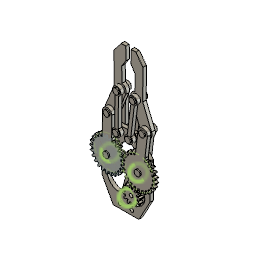
Robotic+Gripper (Autodesk Fusion 360 design; units mm, degrees)
description: Spur Gear; Module: 1.125000; Num Teeth: 24; Pressure Angle: 20.000000; Backlash: 0.00 mm
description: Spur Gear; Module: 1.100000; Num Teeth: 12; Pressure Angle: 20.000000; Backlash: 0.00 mm
Autodesk Fusion 360 part; units mm, degrees
note: some values were not read from the file. Chosen so that the rebuilt part matches the saved one: a direction. Set by a fixed rule: which sketch regions a step uses.
(part 1 of 5)
sketch "Sketch1" plane through (0, 0, 0) normal (0, 0, 1) x (1, 0, 0)
  line L0 (0, -5) -> (22, -5)
  arc A0 (22, -5) -> (22, 5) centre (22, 0) ccw
  line L1 (22, 5) -> (0, 5)
  arc A1 (0, 5) -> (0, -5) centre (0, 0) ccw
  line L2 (0, 0) -> (22, 0) construction
  circle A2 centre (0, 0) radius 1.5
  circle A3 centre (22, 0) radius 1.5
  line L3 (51.4959, 17.929) -> (55.4376, 8.3418)
  line L4 (55.4376, 8.3418) -> (23.9013, -4.6244)
  line L5 (51.4959, 17.929) -> (20.05, 5)
  line L6 (44.0768, 14.8786) -> (53.863, 12.1717)
  line L7 (39.0014, 5.4117) -> (26.978, 0.4683)
  line L8 (39.0014, 5.4117) -> (45.3296, 4.1859)
  dimension "d1" = 22
  dimension "d2" = 10
  dimension "d3" = 3
  dimension "d4" = 3
  dimension "d7" = 1.95
  dimension "d8" = 157.65
  dimension "d9" = 34
  dimension "d10" = 13
  constraint tangent L0 A0
  constraint tangent A0 L1
  constraint parallel L0 L1
  constraint tangent L1 A1
  constraint tangent L0 A1
  constraint horizontal L2
  constraint coincident A1.centre L2.start
  constraint concentric A1 A2
  constraint concentric A0 A3
  constraint coincident A0 L4.end
  constraint tangent A0 L4
  constraint perpendicular L3 L4
  constraint coincident L1 L5.end
  constraint perpendicular L3 L5
  constraint coincident L5 L6.start
  constraint coincident L3 L6.end
  constraint coincident A0 L7.end
  constraint perpendicular L3 L7
  constraint coincident L4 L8.end
  measures "d1" distance of A1.centre A0.centre
  measures "d2" diameter of A0
  measures "d3" diameter of A2
  measures "d4" diameter of A3
  measures "d7" horizontal distance of A0.centre L5.end
  measures "d8" angle of L1 L5
  measures "d9" distance of L3.start L5.end
  measures "d10" distance of L7.start L7.end
extrude "Extrude1" add sketch "Sketch1" along normal blind 3 contours L0 A0 L1 A1 | A0 L1 L3 L4 L5 L6 L7 L8 makes body 1 in component "Gripper (1)"
sketch "Sketch2" plane through (0, 0, 0) normal (0, 0, 1) x (1, 0, 0)
  circle A0 centre (5, 10) radius 1.5
  circle A1 centre (5, 10) radius 3.5
  line L0 (5, 10) -> (36, 10)
  circle A2 centre (36, 10) radius 1.5
  circle A3 centre (36, 10) radius 3.5
  line L1 (8.1623, 11.5) -> (32.8377, 11.5)
  line L2 (8.1623, 8.5) -> (32.8377, 8.5)
  dimension "d13" = 3
  dimension "d14" = 7
  dimension "d15" = 3
  dimension "d16" = 7
  dimension "d17" = 31
  dimension "d18" = 1.5
  constraint concentric A0 A1
  constraint coincident A0.centre A1.centre
  constraint horizontal L0
  constraint coincident L0.end A2.centre
  constraint concentric A2 A3
  constraint coincident A1 L1.start
  constraint coincident A3 L1.end
  constraint horizontal L1
  constraint symmetric L0 L1.start L2.start
  constraint symmetric L0 L1.end L2.end
  measures "d13" diameter of A0
  measures "d14" diameter of A1
  measures "d15" diameter of A2
  measures "d16" diameter of A3
  measures "d17" distance of A0.centre L0.end
  measures "d18" distance of L0 L1
extrude "Extrude1'" add sketch "Sketch2" along normal blind 3 separate body makes body 2 in component "Connecting rod"
sketch "Sketch3" plane through (0, 0, 0) normal (0, 0, 1) x (1, 0, 0)
  line L0 (0, 0) -> (0, 62) construction
  line L1 (0, 62) -> (-7.9898, 62)
  line L2 (-7.9898, 62) -> (-20.5, 47.8997)
  line L3 (-20.5, 47.8997) -> (-20.5, 17.5997)
  line L4 (-11, 0) -> (0, 0)
  line L5 (-20.5, 17.5997) -> (-11, 0)
  circle A0 centre (-5.2398, 58) radius 1.5
  circle A1 centre (-13.5, 37.5997) radius 1.5
  circle A2 centre (-5, 4) radius 1.5
  circle A3 centre (13.5, 37.5997) radius 1.5
  line L6 (20.5, 17.5997) -> (11, 0)
  circle A4 centre (5.2398, 58) radius 1.5
  line L7 (7.9898, 62) -> (20.5, 47.8997)
  line L8 (20.5, 47.8997) -> (20.5, 17.5997)
  line L9 (11, 0) -> (0, 0)
  line L10 (0, 62) -> (7.9898, 62)
  circle A5 centre (5, 4) radius 1.5
  circle A6 centre (7.5, 17.5997) radius 8.5
  line L11 (20.5, 17.5997) -> (0, 17.5997) construction
  dimension "d21" = 62
  dimension "d22" = 11
  dimension "d23" = 20
  dimension "d24" = 20.5
  dimension "d25" = 30.3
  dimension "d26" = 18.85
  dimension "d27" = 3
  dimension "d28" = 4
  dimension "d29" = 2.75
  dimension "d30" = 3
  dimension "d31" = 3
  dimension "d32" = 7
  dimension "d33" = 10.3
  dimension "d34" = 4
  dimension "d35" = 6
  dimension "d36" = 17
  dimension "d37" = 13
  constraint coincident L0.start L4.end
  constraint vertical L0
  constraint perpendicular L0 L1
  constraint perpendicular L1 L3
  constraint perpendicular L0 L4
  constraint symmetric L4.end L0 L9.end
  constraint symmetric L1.start L0 L10.start
  constraint symmetric L0 L1.end L7.start
  constraint symmetric L0 L2.end L7.end
  constraint symmetric L0 L3.end L6.start
  constraint symmetric L0 L4.start L6.end
  constraint symmetric L0 L4.end L9.end
  constraint symmetric L0 A0 A4
  constraint symmetric L0 A1 A3
  constraint symmetric L0 A2 A5
  constraint coincident L0 L11.end
  constraint perpendicular L0 L11
  measures "d21" distance of L0.start L0.end
  measures "d22" distance of L4.start L0.start
  measures "d23" distance of L3.end L4.start
  measures "d24" distance of L0 L3
  measures "d25" distance of L2.end L3.end
  measures "d26" distance of L1.end L2.end
  measures "d27" diameter of A0
  measures "d28" distance of L1 A0.centre
  measures "d29" horizontal distance of L1.end A0.centre
  measures "d30" diameter of A1
  measures "d31" diameter of A2
  measures "d32" distance of L3 A1.centre
  measures "d33" vertical distance of L2.end A1.centre
  measures "d34" distance of L4 A2.centre
  measures "d35" horizontal distance of L4.start A2.centre
  measures "d36" diameter of A6
  measures "d37" distance of L6.start A6.centre
extrude "Extrude1''" add sketch "Sketch3" along normal blind 3 separate body makes body 3 in component "Component"
sketch "Sketch4" plane through (0, 0, 3) normal (0, 0, 1) x (1, 0, 0)
  circle A0 centre (5, 4) radius 1.5
  circle A1 centre (7.5, 17.5997) radius 8.5
  circle A2 centre (-13.5, 37.5997) radius 1.5
  circle A3 centre (-5, 4) radius 1.5
  circle A4 centre (13.5, 37.5997) radius 1.5
  circle A5 centre (5.2398, 58) radius 1.5
  circle A6 centre (-5.2398, 58) radius 1.5
  line L0 (-7.9898, 62) -> (-20.5, 47.8997)
  line L1 (-20.5, 47.8997) -> (-20.5, 17.5997)
  line L2 (-20.5, 17.5997) -> (-11, 0)
  line L3 (-11, 0) -> (11, 0)
  line L4 (11, 0) -> (20.5, 17.5997)
  line L5 (20.5, 17.5997) -> (20.5, 47.8997)
  line L6 (20.5, 47.8997) -> (7.9898, 62)
  line L7 (7.9898, 62) -> (-7.9898, 62)
  spline S0 degree 5 poles (-12.9887, 25.9698) (-12.8812, 26.0083) (-12.6712, 26.1424) (-12.369, 26.5664) (-11.9726, 27.7138) (-11.4084, 30.1864) (-10.6796, 33.5496) (-9.6904, 37.5033) (-8.3597, 41.6551) (-6.6383, 45.5821) (-4.523, 48.8897) (-2.0756, 51.2778) (0.5698, 52.5846) (3.2369, 52.7612) (5.73, 51.8583) (7.8603, 50.0084) (9.4696, 47.4098) (10.4581, 44.3118) (10.8014, 40.9955) (10.5337, 37.7435) (9.7361, 34.8098) (8.5231, 32.3916) (7.0294, 30.5968) (5.398, 29.4192) (3.7666, 28.6961) (2.255, 28.1207) (0.9516, 27.3511) (-0.1001, 26.0957) (-0.9153, 24.2102) (-1.5814, 21.787) (-2.2274, 19.0805) (-2.9952, 16.4345) (-4.0102, 14.2098) (-5.352, 12.7108) (-7.0248, 12.1143) (-8.9268, 12.3927) (-10.8888, 13.3779) (-12.7158, 14.8289) (-14.2263, 16.4978) (-15.2944, 18.1976) (-15.8878, 19.8639) (-16.0433, 21.491) (-15.8437, 23.0636) (-15.3956, 24.5094) (-14.8046, 25.5948) (-14.1624, 26.0841) (-13.6639, 26.001) (-13.3163, 25.9113) (-13.0962, 25.9312) (-12.9887, 25.9698) knots 0 0 0 0 0 0 0.022222 0.044444 0.066667 0.088889 0.111111 0.133333 0.155556 0.177778 0.2 0.222222 0.244444 0.266667 0.288889 0.311111 0.333333 0.355556 0.377778 0.4 0.422222 0.444444 0.466667 0.488889 0.511111 0.533333 0.555556 0.577778 0.6 0.622222 0.644444 0.666667 0.688889 0.711111 0.733333 0.755556 0.777778 0.8 0.822222 0.844444 0.866667 0.888889 0.911111 0.933333 0.955556 0.977778 1 1 1 1 1 1
  point P0 (-5, 47.9245)
  point P1 (9, 47.9245)
  point P2 (6, 29.9245)
  point P3 (-0.0238, 25.9698)
  point P4 (-5.4883, 12.8977)
  point P5 (-14.0601, 16.4336)
  point P6 (-15.6674, 23.5054)
  point P7 (-14.0601, 25.9698)
extrude "Extrude2" cut sketch "Sketch4" against normal blind 3 contours S0 bodies 3 in component "Component"
sketch "Sketch1 (2)" plane through (0, 0, 0) normal (0, 0, 1) x (1, 0, 0) in component "Spur Gear (24 teeth)"
  circle A0 centre (0, 0) radius 12.0992
  circle A1 centre (0, 0) radius 1.5
extrude "Extrude1'''" add sketch "Sketch1 (2)" along normal blind 3 separate body makes body 4 in component "Spur Gear (24 teeth)"
sketch "Sketch2 (2)" plane through (0, 0, 0) normal (0, 0, 1) x (1, 0, 0) in component "Spur Gear (24 teeth)"
  spline S0 degree 5 poles (12.6449, -1.0183) (12.6506, -1.0187) (12.6618, -1.0195) (12.6788, -1.0202) (12.7014, -1.0203) (12.7297, -1.0195) (12.758, -1.0178) (12.7864, -1.0156) (12.8147, -1.0131) (12.8431, -1.0105) (12.8715, -1.0076) (12.8999, -1.0045) (12.9284, -1.0011) (12.9568, -0.9973) (12.9852, -0.9932) (13.0137, -0.9886) (13.0421, -0.9838) (13.0705, -0.9787) (13.099, -0.9733) (13.1274, -0.9678) (13.1559, -0.962) (13.1843, -0.956) (13.2127, -0.9498) (13.2412, -0.9433) (13.2696, -0.9366) (13.298, -0.9297) (13.3264, -0.9226) (13.3549, -0.9152) (13.3833, -0.9076) (13.4117, -0.8999) (13.4401, -0.8919) (13.4684, -0.8838) (13.4968, -0.8754) (13.5252, -0.8669) (13.5535, -0.8581) (13.5819, -0.8492) (13.6102, -0.8401) (13.6385, -0.8308) (13.6669, -0.8214) (13.6952, -0.8117) (13.7234, -0.8019) (13.7517, -0.7919) (13.78, -0.7817) (13.8082, -0.7714) (13.8365, -0.7609) (13.8647, -0.7502) (13.8929, -0.7393) (13.9211, -0.7283) (13.9492, -0.7171) (13.9774, -0.7058) (14.0055, -0.6943) (14.0337, -0.6826) (14.0618, -0.6708) (14.0898, -0.6588) (14.1179, -0.6467) (14.146, -0.6344) (14.174, -0.6219) (14.202, -0.6093) (14.23, -0.5966) (14.2579, -0.5837) (14.2859, -0.5706) (14.3138, -0.5574) (14.3417, -0.544) (14.3696, -0.5305) (14.3975, -0.5169) (14.4253, -0.5031) (14.4531, -0.4891) (14.4809, -0.4751) (14.5087, -0.4608) (14.5364, -0.4465) (14.5641, -0.4319) (14.5863, -0.4202) (14.6029, -0.4114) (14.6139, -0.4054) (14.6195, -0.4024) knots 0 0 0 0 0 0 0.01428571 0.02857143 0.04285714 0.05714286 0.07142857 0.08571429 0.1 0.11428571 0.12857143 0.14285714 0.15714286 0.17142857 0.18571429 0.2 0.21428571 0.22857143 0.24285714 0.25714286 0.27142857 0.28571429 0.3 0.31428571 0.32857143 0.34285714 0.35714286 0.37142857 0.38571429 0.4 0.41428571 0.42857143 0.44285714 0.45714286 0.47142857 0.48571429 0.5 0.51428571 0.52857143 0.54285714 0.55714286 0.57142857 0.58571429 0.6 0.61428571 0.62857143 0.64285714 0.65714286 0.67142857 0.68571429 0.7 0.71428571 0.72857143 0.74285714 0.75714286 0.77142857 0.78571429 0.8 0.81428571 0.82857143 0.84285714 0.85714286 0.87142857 0.88571429 0.9 0.91428571 0.92857143 0.94285714 0.95714286 0.97142857 0.98571429 1 1 1 1 1 1
  spline S1 degree 5 poles (12.6449, 1.0183) (12.6506, 1.0187) (12.6618, 1.0195) (12.6788, 1.0202) (12.7014, 1.0203) (12.7297, 1.0195) (12.758, 1.0178) (12.7864, 1.0156) (12.8147, 1.0131) (12.8431, 1.0105) (12.8715, 1.0076) (12.8999, 1.0045) (12.9284, 1.0011) (12.9568, 0.9973) (12.9852, 0.9932) (13.0137, 0.9886) (13.0421, 0.9838) (13.0705, 0.9787) (13.099, 0.9733) (13.1274, 0.9678) (13.1559, 0.962) (13.1843, 0.956) (13.2127, 0.9498) (13.2412, 0.9433) (13.2696, 0.9366) (13.298, 0.9297) (13.3264, 0.9226) (13.3549, 0.9152) (13.3833, 0.9076) (13.4117, 0.8999) (13.4401, 0.8919) (13.4684, 0.8838) (13.4968, 0.8754) (13.5252, 0.8669) (13.5535, 0.8581) (13.5819, 0.8492) (13.6102, 0.8401) (13.6385, 0.8308) (13.6669, 0.8214) (13.6952, 0.8117) (13.7234, 0.8019) (13.7517, 0.7919) (13.78, 0.7817) (13.8082, 0.7714) (13.8365, 0.7609) (13.8647, 0.7502) (13.8929, 0.7393) (13.9211, 0.7283) (13.9492, 0.7171) (13.9774, 0.7058) (14.0055, 0.6943) (14.0337, 0.6826) (14.0618, 0.6708) (14.0898, 0.6588) (14.1179, 0.6467) (14.146, 0.6344) (14.174, 0.6219) (14.202, 0.6093) (14.23, 0.5966) (14.2579, 0.5837) (14.2859, 0.5706) (14.3138, 0.5574) (14.3417, 0.544) (14.3696, 0.5305) (14.3975, 0.5169) (14.4253, 0.5031) (14.4531, 0.4891) (14.4809, 0.4751) (14.5087, 0.4608) (14.5364, 0.4465) (14.5641, 0.4319) (14.5863, 0.4202) (14.6029, 0.4114) (14.6139, 0.4054) (14.6195, 0.4024) knots 0 0 0 0 0 0 0.01428571 0.02857143 0.04285714 0.05714286 0.07142857 0.08571429 0.1 0.11428571 0.12857143 0.14285714 0.15714286 0.17142857 0.18571429 0.2 0.21428571 0.22857143 0.24285714 0.25714286 0.27142857 0.28571429 0.3 0.31428571 0.32857143 0.34285714 0.35714286 0.37142857 0.38571429 0.4 0.41428571 0.42857143 0.44285714 0.45714286 0.47142857 0.48571429 0.5 0.51428571 0.52857143 0.54285714 0.55714286 0.57142857 0.58571429 0.6 0.61428571 0.62857143 0.64285714 0.65714286 0.67142857 0.68571429 0.7 0.71428571 0.72857143 0.74285714 0.75714286 0.77142857 0.78571429 0.8 0.81428571 0.82857143 0.84285714 0.85714286 0.87142857 0.88571429 0.9 0.91428571 0.92857143 0.94285714 0.95714286 0.97142857 0.98571429 1 1 1 1 1 1
  arc A0 (14.6195, -0.4024) -> (14.6195, 0.4024) centre (0, 0) ccw
  line L0 (12.0502, -0.9712) -> (12.6449, -1.0183)
  line L1 (12.0502, 0.9712) -> (12.6449, 1.0183)
  line L2 (12.0502, -0.9712) -> (12.0502, 0.9712)
  point P0 (12.7841, -1.0157)
  point P1 (12.9241, -1.0016)
  point P2 (13.0647, -0.9797)
  point P3 (13.2057, -0.9513)
  point P4 (13.3469, -0.9172)
  point P5 (13.4884, -0.8779)
  point P6 (13.63, -0.8336)
  point P7 (13.7716, -0.7847)
  point P8 (13.9132, -0.7313)
  point P9 (14.0548, -0.6737)
  point P10 (14.1963, -0.6119)
  point P11 (14.3376, -0.546)
  point P12 (14.4787, -0.4761)
  point P13 (12.7841, 1.0157)
  point P14 (12.9241, 1.0016)
  point P15 (13.0647, 0.9797)
  point P16 (13.2057, 0.9513)
  point P17 (13.3469, 0.9172)
  point P18 (13.4884, 0.8779)
  point P19 (13.63, 0.8336)
  point P20 (13.7716, 0.7847)
  point P21 (13.9132, 0.7313)
  point P22 (14.0548, 0.6737)
  point P23 (14.1963, 0.6119)
  point P24 (14.3376, 0.546)
  point P25 (14.4787, 0.4761)
extrude "Extrude2'" add sketch "Sketch2 (2)" along normal blind 3 bodies 4 in component "Spur Gear (24 teeth)"
fillet "Fillet1" radius 0.1 2 edges at (12.0601, -0.972, 1.5) (12.0601, 0.972, 1.5) on bodies 4 in component "Spur Gear (24 teeth)"
pattern_circular "C-Pattern1" count 24 over 360 about axis through (0, 0, 0) along (0, 0, 1) of "Extrude2'", "Fillet1" in component "Spur Gear (24 teeth)"
sketch "Sketch3 (2)" plane through (0, 0, 0) normal (0, 0, 1) x (1, 0, 0) in component "Spur Gear (24 teeth)"
  circle A0 centre (0, 0) radius 13.5 construction
sketch "Sketch1 (3)" plane through (-40.3607, 8.0279, 6) normal (0, 0, 1) x (0.469472, -0.882948, 0) in component "Component"
  arc A0 (-25.4753, 39.3265) -> (-25.5784, 38.3085) centre (-13.5, 37.5997) ccw
  arc A1 (-25.6831, 38.2145) -> (-25.5784, 38.3085) centre (-25.6782, 38.3144) ccw
  line L0 (-25.6831, 38.2145) -> (-26.1698, 38.2384)
  spline S0 degree 5 poles (-26.1698, 38.2384) (-26.1754, 38.2386) (-26.1867, 38.2391) (-26.2037, 38.2393) (-26.2263, 38.2387) (-26.2545, 38.237) (-26.2828, 38.2345) (-26.3111, 38.2314) (-26.3394, 38.2281) (-26.3677, 38.2246) (-26.396, 38.2209) (-26.4243, 38.217) (-26.4526, 38.2127) (-26.4809, 38.2081) (-26.5092, 38.2031) (-26.5375, 38.1977) (-26.5657, 38.192) (-26.594, 38.186) (-26.6223, 38.1798) (-26.6505, 38.1734) (-26.6788, 38.1668) (-26.707, 38.16) (-26.7353, 38.1529) (-26.7635, 38.1456) (-26.7917, 38.138) (-26.8199, 38.1303) (-26.8481, 38.1223) (-26.8763, 38.114) (-26.9045, 38.1056) (-26.9326, 38.097) (-26.9608, 38.0882) (-26.9889, 38.0792) (-27.017, 38.07) (-27.0451, 38.0607) (-27.0732, 38.0511) (-27.1012, 38.0413) (-27.1293, 38.0313) (-27.1573, 38.0212) (-27.1853, 38.0109) (-27.2133, 38.0004) (-27.2413, 37.9897) (-27.2693, 37.9789) (-27.2972, 37.9679) (-27.3251, 37.9567) (-27.3531, 37.9453) (-27.3809, 37.9338) (-27.4088, 37.9221) (-27.4366, 37.9103) (-27.4645, 37.8982) (-27.4923, 37.8861) (-27.5201, 37.8737) (-27.5478, 37.8612) (-27.5755, 37.8486) (-27.6033, 37.8357) (-27.6309, 37.8228) (-27.6586, 37.8096) (-27.6863, 37.7963) (-27.7139, 37.7829) (-27.7415, 37.7693) (-27.769, 37.7556) (-27.7966, 37.7417) (-27.8241, 37.7277) (-27.8516, 37.7135) (-27.879, 37.6991) (-27.9065, 37.6847) (-27.9339, 37.67) (-27.9613, 37.6553) (-27.9886, 37.6403) (-28.0159, 37.6253) (-28.0432, 37.6101) (-28.0705, 37.5948) (-28.0923, 37.5824) (-28.1086, 37.573) (-28.1195, 37.5668) (-28.125, 37.5636) knots 0 0 0 0 0 0 0.01428571 0.02857143 0.04285714 0.05714286 0.07142857 0.08571429 0.1 0.11428571 0.12857143 0.14285714 0.15714286 0.17142857 0.18571429 0.2 0.21428571 0.22857143 0.24285714 0.25714286 0.27142857 0.28571429 0.3 0.31428571 0.32857143 0.34285714 0.35714286 0.37142857 0.38571429 0.4 0.41428571 0.42857143 0.44285714 0.45714286 0.47142857 0.48571429 0.5 0.51428571 0.52857143 0.54285714 0.55714286 0.57142857 0.58571429 0.6 0.61428571 0.62857143 0.64285714 0.65714286 0.67142857 0.68571429 0.7 0.71428571 0.72857143 0.74285714 0.75714286 0.77142857 0.78571429 0.8 0.81428571 0.82857143 0.84285714 0.85714286 0.87142857 0.88571429 0.9 0.91428571 0.92857143 0.94285714 0.95714286 0.97142857 0.98571429 1 1 1 1 1 1
  arc A2 (-28.125, 37.5636) -> (-28.1008, 36.7591) centre (-13.5, 37.5997) ccw
  spline S1 degree 5 poles (-28.1008, 36.7591) (-28.0952, 36.7563) (-28.084, 36.7507) (-28.0671, 36.7423) (-28.0446, 36.7313) (-28.0165, 36.7176) (-27.9883, 36.7041) (-27.9601, 36.6907) (-27.9319, 36.6774) (-27.9037, 36.6643) (-27.8755, 36.6514) (-27.8472, 36.6386) (-27.819, 36.6259) (-27.7907, 36.6134) (-27.7624, 36.601) (-27.734, 36.5888) (-27.7057, 36.5767) (-27.6773, 36.5648) (-27.649, 36.5531) (-27.6206, 36.5415) (-27.5922, 36.53) (-27.5638, 36.5187) (-27.5353, 36.5076) (-27.5069, 36.4966) (-27.4784, 36.4858) (-27.4499, 36.4751) (-27.4215, 36.4646) (-27.393, 36.4543) (-27.3645, 36.4442) (-27.336, 36.4342) (-27.3074, 36.4243) (-27.2789, 36.4147) (-27.2503, 36.4052) (-27.2218, 36.3958) (-27.1932, 36.3867) (-27.1647, 36.3777) (-27.1361, 36.3689) (-27.1075, 36.3603) (-27.0789, 36.3519) (-27.0503, 36.3436) (-27.0217, 36.3356) (-26.9931, 36.3277) (-26.9645, 36.32) (-26.9359, 36.3125) (-26.9073, 36.3052) (-26.8786, 36.2981) (-26.85, 36.2912) (-26.8214, 36.2845) (-26.7928, 36.278) (-26.7642, 36.2717) (-26.7355, 36.2656) (-26.7069, 36.2598) (-26.6783, 36.2542) (-26.6497, 36.2488) (-26.6211, 36.2437) (-26.5925, 36.2388) (-26.5639, 36.2341) (-26.5353, 36.2296) (-26.5067, 36.2253) (-26.4782, 36.2213) (-26.4496, 36.2176) (-26.4211, 36.2143) (-26.3925, 36.2114) (-26.364, 36.2088) (-26.3355, 36.2066) (-26.3071, 36.2046) (-26.2786, 36.2028) (-26.2502, 36.2012) (-26.2218, 36.1999) (-26.1934, 36.199) (-26.1651, 36.199) (-26.1425, 36.1998) (-26.1256, 36.201) (-26.1143, 36.2021) (-26.1087, 36.2028) knots -1 -1 -1 -1 -1 -1 -0.98571429 -0.97142857 -0.95714286 -0.94285714 -0.92857143 -0.91428571 -0.9 -0.88571429 -0.87142857 -0.85714286 -0.84285714 -0.82857143 -0.81428571 -0.8 -0.78571429 -0.77142857 -0.75714286 -0.74285714 -0.72857143 -0.71428571 -0.7 -0.68571429 -0.67142857 -0.65714286 -0.64285714 -0.62857143 -0.61428571 -0.6 -0.58571429 -0.57142857 -0.55714286 -0.54285714 -0.52857143 -0.51428571 -0.5 -0.48571429 -0.47142857 -0.45714286 -0.44285714 -0.42857143 -0.41428571 -0.4 -0.38571429 -0.37142857 -0.35714286 -0.34285714 -0.32857143 -0.31428571 -0.3 -0.28571429 -0.27142857 -0.25714286 -0.24285714 -0.22857143 -0.21428571 -0.2 -0.18571429 -0.17142857 -0.15714286 -0.14285714 -0.12857143 -0.11428571 -0.1 -0.08571429 -0.07142857 -0.05714286 -0.04285714 -0.02857143 -0.01428571 0 0 0 0 0 0
  line L1 (-26.1087, 36.2028) -> (-25.6244, 36.2558)
  arc A3 (-25.5142, 36.1682) -> (-25.6244, 36.2558) centre (-25.6135, 36.1563) ccw
  arc A4 (-25.5142, 36.1682) -> (-25.3503, 35.1582) centre (-13.5, 37.5997) ccw
  arc A5 (-25.4271, 35.0403) -> (-25.3503, 35.1582) centre (-25.4483, 35.1381) ccw
  line L2 (-25.4271, 35.0403) -> (-25.9033, 34.9374)
  spline S2 degree 5 poles (-25.9033, 34.9374) (-25.9089, 34.9362) (-25.9199, 34.9337) (-25.9363, 34.9295) (-25.958, 34.9232) (-25.9849, 34.9142) (-26.0115, 34.9044) (-26.0381, 34.8942) (-26.0645, 34.8836) (-26.0909, 34.8729) (-26.1173, 34.862) (-26.1437, 34.8509) (-26.1699, 34.8395) (-26.196, 34.8277) (-26.222, 34.8155) (-26.248, 34.803) (-26.2738, 34.7901) (-26.2996, 34.7771) (-26.3253, 34.7638) (-26.3509, 34.7503) (-26.3765, 34.7366) (-26.402, 34.7226) (-26.4275, 34.7085) (-26.4528, 34.6941) (-26.4781, 34.6796) (-26.5034, 34.6647) (-26.5285, 34.6497) (-26.5536, 34.6345) (-26.5787, 34.6191) (-26.6036, 34.6035) (-26.6285, 34.5877) (-26.6534, 34.5717) (-26.6781, 34.5556) (-26.7029, 34.5392) (-26.7275, 34.5227) (-26.7521, 34.506) (-26.7766, 34.4891) (-26.8011, 34.4721) (-26.8254, 34.4549) (-26.8498, 34.4375) (-26.874, 34.4199) (-26.8982, 34.4022) (-26.9224, 34.3844) (-26.9465, 34.3663) (-26.9705, 34.3481) (-26.9944, 34.3298) (-27.0183, 34.3113) (-27.0421, 34.2926) (-27.0659, 34.2738) (-27.0896, 34.2548) (-27.1132, 34.2357) (-27.1368, 34.2165) (-27.1603, 34.1971) (-27.1838, 34.1775) (-27.2072, 34.1578) (-27.2305, 34.138) (-27.2538, 34.118) (-27.277, 34.0978) (-27.3001, 34.0776) (-27.3232, 34.0572) (-27.3462, 34.0366) (-27.3691, 34.0159) (-27.392, 33.9951) (-27.4148, 33.9742) (-27.4376, 33.9531) (-27.4603, 33.9319) (-27.4829, 33.9105) (-27.5055, 33.889) (-27.5279, 33.8674) (-27.5504, 33.8457) (-27.5727, 33.8238) (-27.5906, 33.8062) (-27.6039, 33.7929) (-27.6128, 33.7841) (-27.6173, 33.7796) knots 0 0 0 0 0 0 0.01428571 0.02857143 0.04285714 0.05714286 0.07142857 0.08571429 0.1 0.11428571 0.12857143 0.14285714 0.15714286 0.17142857 0.18571429 0.2 0.21428571 0.22857143 0.24285714 0.25714286 0.27142857 0.28571429 0.3 0.31428571 0.32857143 0.34285714 0.35714286 0.37142857 0.38571429 0.4 0.41428571 0.42857143 0.44285714 0.45714286 0.47142857 0.48571429 0.5 0.51428571 0.52857143 0.54285714 0.55714286 0.57142857 0.58571429 0.6 0.61428571 0.62857143 0.64285714 0.65714286 0.67142857 0.68571429 0.7 0.71428571 0.72857143 0.74285714 0.75714286 0.77142857 0.78571429 0.8 0.81428571 0.82857143 0.84285714 0.85714286 0.87142857 0.88571429 0.9 0.91428571 0.92857143 0.94285714 0.95714286 0.97142857 0.98571429 1 1 1 1 1 1
  arc A6 (-27.6173, 33.7796) -> (-27.3857, 33.0088) centre (-13.5, 37.5997) ccw
  spline S3 degree 5 poles (-27.3857, 33.0088) (-27.3796, 33.0075) (-27.3673, 33.005) (-27.3488, 33.0013) (-27.3242, 32.9964) (-27.2935, 32.9905) (-27.2628, 32.9847) (-27.2321, 32.9791) (-27.2015, 32.9736) (-27.1708, 32.9682) (-27.1402, 32.963) (-27.1096, 32.958) (-27.079, 32.9531) (-27.0484, 32.9483) (-27.0179, 32.9437) (-26.9874, 32.9392) (-26.9569, 32.9349) (-26.9264, 32.9307) (-26.896, 32.9267) (-26.8655, 32.9229) (-26.8351, 32.9191) (-26.8048, 32.9156) (-26.7744, 32.9122) (-26.7441, 32.909) (-26.7138, 32.9059) (-26.6836, 32.903) (-26.6533, 32.9002) (-26.6231, 32.8976) (-26.593, 32.8951) (-26.5628, 32.8929) (-26.5327, 32.8907) (-26.5027, 32.8888) (-26.4726, 32.887) (-26.4426, 32.8854) (-26.4127, 32.884) (-26.3828, 32.8827) (-26.3529, 32.8816) (-26.3231, 32.8807) (-26.2933, 32.8799) (-26.2635, 32.8793) (-26.2338, 32.879) (-26.2041, 32.8787) (-26.1745, 32.8787) (-26.1449, 32.8789) (-26.1154, 32.8793) (-26.0859, 32.8798) (-26.0565, 32.8805) (-26.0271, 32.8815) (-25.9978, 32.8826) (-25.9685, 32.8839) (-25.9393, 32.8855) (-25.9101, 32.8872) (-25.881, 32.8892) (-25.852, 32.8914) (-25.823, 32.8939) (-25.7941, 32.8965) (-25.7653, 32.8994) (-25.7365, 32.9025) (-25.7078, 32.9058) (-25.6792, 32.9093) (-25.6507, 32.9131) (-25.6222, 32.9173) (-25.5939, 32.9219) (-25.5657, 32.9268) (-25.5376, 32.932) (-25.5096, 32.9374) (-25.4816, 32.9431) (-25.4538, 32.9489) (-25.426, 32.9549) (-25.3984, 32.9615) (-25.371, 32.9687) (-25.3494, 32.9754) (-25.3334, 32.981) (-25.3228, 32.9849) (-25.3175, 32.987) knots -1 -1 -1 -1 -1 -1 -0.98571429 -0.97142857 -0.95714286 -0.94285714 -0.92857143 -0.91428571 -0.9 -0.88571429 -0.87142857 -0.85714286 -0.84285714 -0.82857143 -0.81428571 -0.8 -0.78571429 -0.77142857 -0.75714286 -0.74285714 -0.72857143 -0.71428571 -0.7 -0.68571429 -0.67142857 -0.65714286 -0.64285714 -0.62857143 -0.61428571 -0.6 -0.58571429 -0.57142857 -0.55714286 -0.54285714 -0.52857143 -0.51428571 -0.5 -0.48571429 -0.47142857 -0.45714286 -0.44285714 -0.42857143 -0.41428571 -0.4 -0.38571429 -0.37142857 -0.35714286 -0.34285714 -0.32857143 -0.31428571 -0.3 -0.28571429 -0.27142857 -0.25714286 -0.24285714 -0.22857143 -0.21428571 -0.2 -0.18571429 -0.17142857 -0.15714286 -0.14285714 -0.12857143 -0.11428571 -0.1 -0.08571429 -0.07142857 -0.05714286 -0.04285714 -0.02857143 -0.01428571 0 0 0 0 0 0
  line L3 (-25.3175, 32.987) -> (-24.8634, 33.1635)
  arc A7 (-24.7343, 33.1074) -> (-24.8634, 33.1635) centre (-24.8272, 33.0703) ccw
  arc A8 (-24.7343, 33.1074) -> (-24.3146, 32.1743) centre (-13.5, 37.5997) ccw
  arc A9 (-24.3583, 32.0406) -> (-24.3146, 32.1743) centre (-24.404, 32.1295) ccw
  line L4 (-24.3583, 32.0406) -> (-24.7917, 31.8179)
  spline S4 degree 5 poles (-24.7917, 31.8179) (-24.7967, 31.8153) (-24.8067, 31.81) (-24.8215, 31.8017) (-24.8408, 31.79) (-24.8644, 31.7744) (-24.8876, 31.758) (-24.9106, 31.7413) (-24.9334, 31.7243) (-24.9562, 31.7071) (-24.9788, 31.6897) (-25.0014, 31.6722) (-25.0238, 31.6543) (-25.046, 31.6361) (-25.0679, 31.6176) (-25.0897, 31.5988) (-25.1114, 31.5798) (-25.1329, 31.5605) (-25.1543, 31.541) (-25.1755, 31.5213) (-25.1967, 31.5014) (-25.2178, 31.4814) (-25.2387, 31.4612) (-25.2595, 31.4407) (-25.2801, 31.4201) (-25.3007, 31.3992) (-25.3211, 31.3782) (-25.3414, 31.357) (-25.3616, 31.3356) (-25.3816, 31.3141) (-25.4016, 31.2924) (-25.4215, 31.2705) (-25.4412, 31.2485) (-25.4609, 31.2264) (-25.4804, 31.204) (-25.4998, 31.1815) (-25.5191, 31.1589) (-25.5383, 31.1361) (-25.5574, 31.1131) (-25.5764, 31.0901) (-25.5953, 31.0668) (-25.6141, 31.0435) (-25.6328, 31.0199) (-25.6514, 30.9963) (-25.6699, 30.9725) (-25.6883, 30.9486) (-25.7066, 30.9245) (-25.7248, 30.9003) (-25.7429, 30.876) (-25.7608, 30.8516) (-25.7787, 30.827) (-25.7965, 30.8023) (-25.8142, 30.7774) (-25.8318, 30.7525) (-25.8493, 30.7274) (-25.8667, 30.7022) (-25.884, 30.6769) (-25.9012, 30.6514) (-25.9183, 30.6259) (-25.9353, 30.6002) (-25.9522, 30.5744) (-25.969, 30.5485) (-25.9857, 30.5224) (-26.0023, 30.4963) (-26.0188, 30.47) (-26.0353, 30.4437) (-26.0516, 30.4172) (-26.0678, 30.3906) (-26.084, 30.3639) (-26.1, 30.3371) (-26.116, 30.3102) (-26.1286, 30.2885) (-26.1381, 30.2723) (-26.1444, 30.2614) (-26.1475, 30.256) knots 0 0 0 0 0 0 0.01428571 0.02857143 0.04285714 0.05714286 0.07142857 0.08571429 0.1 0.11428571 0.12857143 0.14285714 0.15714286 0.17142857 0.18571429 0.2 0.21428571 0.22857143 0.24285714 0.25714286 0.27142857 0.28571429 0.3 0.31428571 0.32857143 0.34285714 0.35714286 0.37142857 0.38571429 0.4 0.41428571 0.42857143 0.44285714 0.45714286 0.47142857 0.48571429 0.5 0.51428571 0.52857143 0.54285714 0.55714286 0.57142857 0.58571429 0.6 0.61428571 0.62857143 0.64285714 0.65714286 0.67142857 0.68571429 0.7 0.71428571 0.72857143 0.74285714 0.75714286 0.77142857 0.78571429 0.8 0.81428571 0.82857143 0.84285714 0.85714286 0.87142857 0.88571429 0.9 0.91428571 0.92857143 0.94285714 0.95714286 0.97142857 0.98571429 1 1 1 1 1 1
  arc A10 (-26.1475, 30.256) -> (-25.7244, 29.5713) centre (-13.5, 37.5997) ccw
  spline S5 degree 5 poles (-25.7244, 29.5713) (-25.7181, 29.5717) (-25.7056, 29.5724) (-25.6868, 29.5736) (-25.6618, 29.5753) (-25.6306, 29.5775) (-25.5994, 29.5799) (-25.5683, 29.5824) (-25.5373, 29.585) (-25.5063, 29.5878) (-25.4754, 29.5907) (-25.4445, 29.5937) (-25.4137, 29.5969) (-25.3829, 29.6002) (-25.3522, 29.6036) (-25.3216, 29.6072) (-25.291, 29.6109) (-25.2605, 29.6148) (-25.23, 29.6188) (-25.1996, 29.623) (-25.1693, 29.6272) (-25.1391, 29.6317) (-25.1089, 29.6362) (-25.0788, 29.641) (-25.0487, 29.6458) (-25.0187, 29.6508) (-24.9888, 29.656) (-24.959, 29.6613) (-24.9292, 29.6667) (-24.8995, 29.6723) (-24.8699, 29.6781) (-24.8403, 29.684) (-24.8109, 29.69) (-24.7815, 29.6962) (-24.7522, 29.7026) (-24.7229, 29.7091) (-24.6938, 29.7158) (-24.6647, 29.7226) (-24.6358, 29.7296) (-24.6069, 29.7368) (-24.5781, 29.7441) (-24.5493, 29.7515) (-24.5207, 29.7592) (-24.4922, 29.767) (-24.4638, 29.775) (-24.4354, 29.7832) (-24.4072, 29.7915) (-24.3791, 29.8) (-24.351, 29.8087) (-24.3231, 29.8175) (-24.2953, 29.8266) (-24.2676, 29.8358) (-24.24, 29.8453) (-24.2125, 29.8549) (-24.1852, 29.8648) (-24.158, 29.8748) (-24.1308, 29.8851) (-24.1038, 29.8955) (-24.077, 29.9061) (-24.0502, 29.9169) (-24.0237, 29.928) (-23.9973, 29.9394) (-23.9711, 29.9511) (-23.9451, 29.9632) (-23.9193, 29.9755) (-23.8937, 29.988) (-23.8681, 30.0006) (-23.8427, 30.0135) (-23.8174, 30.0265) (-23.7925, 30.04) (-23.7679, 30.0541) (-23.7488, 30.0661) (-23.7347, 30.0756) (-23.7255, 30.0822) (-23.721, 30.0856) knots -1 -1 -1 -1 -1 -1 -0.98571429 -0.97142857 -0.95714286 -0.94285714 -0.92857143 -0.91428571 -0.9 -0.88571429 -0.87142857 -0.85714286 -0.84285714 -0.82857143 -0.81428571 -0.8 -0.78571429 -0.77142857 -0.75714286 -0.74285714 -0.72857143 -0.71428571 -0.7 -0.68571429 -0.67142857 -0.65714286 -0.64285714 -0.62857143 -0.61428571 -0.6 -0.58571429 -0.57142857 -0.55714286 -0.54285714 -0.52857143 -0.51428571 -0.5 -0.48571429 -0.47142857 -0.45714286 -0.44285714 -0.42857143 -0.41428571 -0.4 -0.38571429 -0.37142857 -0.35714286 -0.34285714 -0.32857143 -0.31428571 -0.3 -0.28571429 -0.27142857 -0.25714286 -0.24285714 -0.22857143 -0.21428571 -0.2 -0.18571429 -0.17142857 -0.15714286 -0.14285714 -0.12857143 -0.11428571 -0.1 -0.08571429 -0.07142857 -0.05714286 -0.04285714 -0.02857143 -0.01428571 0 0 0 0 0 0
  line L5 (-23.721, 30.0856) -> (-23.328, 30.3736)
  arc A11 (-23.1888, 30.3529) -> (-23.328, 30.3736) centre (-23.2689, 30.293) ccw
  arc A12 (-23.1888, 30.3529) -> (-22.5419, 29.5602) centre (-13.5, 37.5997) ccw
  arc A13 (-22.5495, 29.4196) -> (-22.5419, 29.5602) centre (-22.6167, 29.4937) ccw
  line L6 (-22.5495, 29.4196) -> (-22.9105, 29.0924)
  spline S6 degree 5 poles (-22.9105, 29.0924) (-22.9147, 29.0886) (-22.9229, 29.0809) (-22.9351, 29.0691) (-22.9507, 29.0527) (-22.9695, 29.0315) (-22.9876, 29.0098) (-23.0055, 28.9876) (-23.0232, 28.9653) (-23.0407, 28.9428) (-23.0581, 28.9202) (-23.0753, 28.8974) (-23.0923, 28.8743) (-23.109, 28.851) (-23.1255, 28.8275) (-23.1417, 28.8037) (-23.1577, 28.7796) (-23.1734, 28.7554) (-23.189, 28.7311) (-23.2045, 28.7066) (-23.2198, 28.6819) (-23.2349, 28.6571) (-23.2499, 28.6321) (-23.2647, 28.607) (-23.2793, 28.5817) (-23.2938, 28.5563) (-23.308, 28.5307) (-23.3222, 28.5049) (-23.3361, 28.4791) (-23.3499, 28.4531) (-23.3636, 28.427) (-23.3771, 28.4007) (-23.3905, 28.3743) (-23.4038, 28.3478) (-23.4168, 28.3212) (-23.4298, 28.2944) (-23.4426, 28.2676) (-23.4552, 28.2406) (-23.4677, 28.2135) (-23.4801, 28.1863) (-23.4924, 28.1589) (-23.5045, 28.1315) (-23.5164, 28.1039) (-23.5283, 28.0763) (-23.54, 28.0485) (-23.5515, 28.0207) (-23.563, 27.9927) (-23.5743, 27.9646) (-23.5855, 27.9364) (-23.5965, 27.9082) (-23.6074, 27.8798) (-23.6182, 27.8513) (-23.6289, 27.8228) (-23.6394, 27.7941) (-23.6498, 27.7653) (-23.6601, 27.7365) (-23.6702, 27.7076) (-23.6803, 27.6785) (-23.6902, 27.6494) (-23.6999, 27.6202) (-23.7096, 27.5909) (-23.7191, 27.5615) (-23.7285, 27.5321) (-23.7378, 27.5025) (-23.747, 27.4729) (-23.756, 27.4431) (-23.7649, 27.4133) (-23.7737, 27.3834) (-23.7824, 27.3535) (-23.791, 27.3234) (-23.7994, 27.2933) (-23.8061, 27.2691) (-23.811, 27.251) (-23.8143, 27.2388) (-23.8159, 27.2328) knots 0 0 0 0 0 0 0.01428571 0.02857143 0.04285714 0.05714286 0.07142857 0.08571429 0.1 0.11428571 0.12857143 0.14285714 0.15714286 0.17142857 0.18571429 0.2 0.21428571 0.22857143 0.24285714 0.25714286 0.27142857 0.28571429 0.3 0.31428571 0.32857143 0.34285714 0.35714286 0.37142857 0.38571429 0.4 0.41428571 0.42857143 0.44285714 0.45714286 0.47142857 0.48571429 0.5 0.51428571 0.52857143 0.54285714 0.55714286 0.57142857 0.58571429 0.6 0.61428571 0.62857143 0.64285714 0.65714286 0.67142857 0.68571429 0.7 0.71428571 0.72857143 0.74285714 0.75714286 0.77142857 0.78571429 0.8 0.81428571 0.82857143 0.84285714 0.85714286 0.87142857 0.88571429 0.9 0.91428571 0.92857143 0.94285714 0.95714286 0.97142857 0.98571429 1 1 1 1 1 1
  arc A14 (-23.8159, 27.2328) -> (-23.2299, 26.681) centre (-13.5, 37.5997) ccw
  spline S7 degree 5 poles (-23.2299, 26.681) (-23.224, 26.6829) (-23.2121, 26.6869) (-23.1942, 26.693) (-23.1705, 26.701) (-23.1409, 26.7113) (-23.1115, 26.7216) (-23.0821, 26.7321) (-23.0528, 26.7426) (-23.0235, 26.7533) (-22.9944, 26.7641) (-22.9654, 26.7751) (-22.9364, 26.7861) (-22.9076, 26.7972) (-22.8788, 26.8085) (-22.8502, 26.8199) (-22.8216, 26.8314) (-22.7931, 26.8431) (-22.7647, 26.8548) (-22.7365, 26.8667) (-22.7083, 26.8787) (-22.6802, 26.8908) (-22.6522, 26.903) (-22.6243, 26.9153) (-22.5966, 26.9278) (-22.5689, 26.9404) (-22.5413, 26.9531) (-22.5139, 26.966) (-22.4866, 26.979) (-22.4593, 26.992) (-22.4322, 27.0053) (-22.4052, 27.0186) (-22.3783, 27.0321) (-22.3515, 27.0457) (-22.3248, 27.0594) (-22.2983, 27.0733) (-22.2719, 27.0873) (-22.2456, 27.1014) (-22.2194, 27.1156) (-22.1933, 27.13) (-22.1674, 27.1445) (-22.1416, 27.1592) (-22.1159, 27.174) (-22.0904, 27.1889) (-22.065, 27.204) (-22.0398, 27.2192) (-22.0146, 27.2346) (-21.9897, 27.2501) (-21.9648, 27.2657) (-21.9401, 27.2815) (-21.9156, 27.2974) (-21.8912, 27.3135) (-21.867, 27.3298) (-21.843, 27.3462) (-21.8191, 27.3628) (-21.7955, 27.3796) (-21.7719, 27.3965) (-21.7485, 27.4135) (-21.7253, 27.4307) (-21.7023, 27.4481) (-21.6795, 27.4657) (-21.6569, 27.4835) (-21.6347, 27.5016) (-21.6127, 27.52) (-21.591, 27.5385) (-21.5695, 27.5573) (-21.5481, 27.5761) (-21.5268, 27.5951) (-21.5058, 27.6142) (-21.4851, 27.6337) (-21.4651, 27.6537) (-21.4497, 27.6702) (-21.4386, 27.6831) (-21.4314, 27.6918) (-21.4279, 27.6962) knots -1 -1 -1 -1 -1 -1 -0.98571429 -0.97142857 -0.95714286 -0.94285714 -0.92857143 -0.91428571 -0.9 -0.88571429 -0.87142857 -0.85714286 -0.84285714 -0.82857143 -0.81428571 -0.8 -0.78571429 -0.77142857 -0.75714286 -0.74285714 -0.72857143 -0.71428571 -0.7 -0.68571429 -0.67142857 -0.65714286 -0.64285714 -0.62857143 -0.61428571 -0.6 -0.58571429 -0.57142857 -0.55714286 -0.54285714 -0.52857143 -0.51428571 -0.5 -0.48571429 -0.47142857 -0.45714286 -0.44285714 -0.42857143 -0.41428571 -0.4 -0.38571429 -0.37142857 -0.35714286 -0.34285714 -0.32857143 -0.31428571 -0.3 -0.28571429 -0.27142857 -0.25714286 -0.24285714 -0.22857143 -0.21428571 -0.2 -0.18571429 -0.17142857 -0.15714286 -0.14285714 -0.12857143 -0.11428571 -0.1 -0.08571429 -0.07142857 -0.05714286 -0.04285714 -0.02857143 -0.01428571 0 0 0 0 0 0
  line L7 (-21.4279, 27.6962) -> (-21.1229, 28.0762)
  arc A15 (-20.9831, 28.0921) -> (-21.1229, 28.0762) centre (-21.0449, 28.0136) ccw
  arc A16 (-20.9831, 28.0921) -> (-20.153, 27.4939) centre (-13.5, 37.5997) ccw
  arc A17 (-20.124, 27.3562) -> (-20.153, 27.4939) centre (-20.208, 27.4104) ccw
  line L8 (-20.124, 27.3562) -> (-20.388, 26.9467)
  spline S8 degree 5 poles (-20.388, 26.9467) (-20.391, 26.9419) (-20.397, 26.9324) (-20.4057, 26.9178) (-20.4166, 26.898) (-20.4292, 26.8726) (-20.4411, 26.8469) (-20.4526, 26.8209) (-20.4639, 26.7947) (-20.475, 26.7685) (-20.486, 26.7421) (-20.4967, 26.7156) (-20.5072, 26.689) (-20.5173, 26.6621) (-20.5271, 26.6351) (-20.5366, 26.6079) (-20.5458, 26.5806) (-20.5547, 26.5531) (-20.5635, 26.5255) (-20.5721, 26.4979) (-20.5805, 26.4701) (-20.5887, 26.4422) (-20.5967, 26.4142) (-20.6045, 26.3861) (-20.6121, 26.3579) (-20.6194, 26.3296) (-20.6266, 26.3012) (-20.6336, 26.2727) (-20.6404, 26.2441) (-20.647, 26.2154) (-20.6534, 26.1866) (-20.6597, 26.1578) (-20.6658, 26.1288) (-20.6717, 26.0998) (-20.6775, 26.0707) (-20.683, 26.0415) (-20.6885, 26.0122) (-20.6937, 25.9829) (-20.6988, 25.9535) (-20.7037, 25.924) (-20.7084, 25.8944) (-20.713, 25.8648) (-20.7175, 25.8351) (-20.7217, 25.8053) (-20.7258, 25.7754) (-20.7298, 25.7455) (-20.7336, 25.7155) (-20.7373, 25.6855) (-20.7408, 25.6554) (-20.7441, 25.6252) (-20.7473, 25.595) (-20.7504, 25.5647) (-20.7533, 25.5344) (-20.756, 25.5039) (-20.7586, 25.4735) (-20.7611, 25.443) (-20.7634, 25.4124) (-20.7656, 25.3817) (-20.7676, 25.3511) (-20.7695, 25.3203) (-20.7712, 25.2895) (-20.7728, 25.2587) (-20.7743, 25.2278) (-20.7756, 25.1968) (-20.7768, 25.1658) (-20.7778, 25.1348) (-20.7787, 25.1037) (-20.7795, 25.0725) (-20.7801, 25.0413) (-20.7806, 25.0101) (-20.781, 24.9788) (-20.7811, 24.9537) (-20.7812, 24.9349) (-20.7812, 24.9224) (-20.7812, 24.9161) knots 0 0 0 0 0 0 0.01428571 0.02857143 0.04285714 0.05714286 0.07142857 0.08571429 0.1 0.11428571 0.12857143 0.14285714 0.15714286 0.17142857 0.18571429 0.2 0.21428571 0.22857143 0.24285714 0.25714286 0.27142857 0.28571429 0.3 0.31428571 0.32857143 0.34285714 0.35714286 0.37142857 0.38571429 0.4 0.41428571 0.42857143 0.44285714 0.45714286 0.47142857 0.48571429 0.5 0.51428571 0.52857143 0.54285714 0.55714286 0.57142857 0.58571429 0.6 0.61428571 0.62857143 0.64285714 0.65714286 0.67142857 0.68571429 0.7 0.71428571 0.72857143 0.74285714 0.75714286 0.77142857 0.78571429 0.8 0.81428571 0.82857143 0.84285714 0.85714286 0.87142857 0.88571429 0.9 0.91428571 0.92857143 0.94285714 0.95714286 0.97142857 0.98571429 1 1 1 1 1 1
  arc A18 (-20.7812, 24.9161) -> (-20.0724, 24.5347) centre (-13.5, 37.5997) ccw
  spline S9 degree 5 poles (-20.0724, 24.5347) (-20.0672, 24.5382) (-20.0567, 24.5451) (-20.041, 24.5555) (-20.0202, 24.5695) (-19.9943, 24.587) (-19.9685, 24.6046) (-19.9428, 24.6223) (-19.9172, 24.6401) (-19.8918, 24.658) (-19.8664, 24.676) (-19.8412, 24.6941) (-19.8161, 24.7122) (-19.7911, 24.7305) (-19.7663, 24.7488) (-19.7415, 24.7672) (-19.7169, 24.7857) (-19.6924, 24.8043) (-19.6681, 24.823) (-19.6438, 24.8418) (-19.6197, 24.8607) (-19.5957, 24.8797) (-19.5719, 24.8987) (-19.5481, 24.9179) (-19.5245, 24.9371) (-19.5011, 24.9564) (-19.4777, 24.9758) (-19.4545, 24.9954) (-19.4315, 25.015) (-19.4086, 25.0346) (-19.3858, 25.0544) (-19.3632, 25.0743) (-19.3407, 25.0943) (-19.3183, 25.1144) (-19.2961, 25.1345) (-19.2741, 25.1548) (-19.2521, 25.1751) (-19.2304, 25.1956) (-19.2088, 25.2161) (-19.1873, 25.2368) (-19.1661, 25.2575) (-19.1449, 25.2783) (-19.124, 25.2993) (-19.1032, 25.3203) (-19.0826, 25.3414) (-19.0621, 25.3627) (-19.0418, 25.384) (-19.0217, 25.4054) (-19.0017, 25.427) (-18.982, 25.4486) (-18.9624, 25.4703) (-18.943, 25.4922) (-18.9239, 25.5142) (-18.9049, 25.5363) (-18.8862, 25.5585) (-18.8676, 25.5808) (-18.8493, 25.6032) (-18.8311, 25.6257) (-18.8131, 25.6484) (-18.7954, 25.6711) (-18.7779, 25.694) (-18.7607, 25.7171) (-18.7439, 25.7403) (-18.7275, 25.7637) (-18.7113, 25.7872) (-18.6953, 25.8109) (-18.6795, 25.8347) (-18.6639, 25.8585) (-18.6486, 25.8824) (-18.6337, 25.9066) (-18.6195, 25.9311) (-18.6089, 25.9511) (-18.6015, 25.9663) (-18.5968, 25.9766) (-18.5945, 25.9818) knots -1 -1 -1 -1 -1 -1 -0.98571429 -0.97142857 -0.95714286 -0.94285714 -0.92857143 -0.91428571 -0.9 -0.88571429 -0.87142857 -0.85714286 -0.84285714 -0.82857143 -0.81428571 -0.8 -0.78571429 -0.77142857 -0.75714286 -0.74285714 -0.72857143 -0.71428571 -0.7 -0.68571429 -0.67142857 -0.65714286 -0.64285714 -0.62857143 -0.61428571 -0.6 -0.58571429 -0.57142857 -0.55714286 -0.54285714 -0.52857143 -0.51428571 -0.5 -0.48571429 -0.47142857 -0.45714286 -0.44285714 -0.42857143 -0.41428571 -0.4 -0.38571429 -0.37142857 -0.35714286 -0.34285714 -0.32857143 -0.31428571 -0.3 -0.28571429 -0.27142857 -0.25714286 -0.24285714 -0.22857143 -0.21428571 -0.2 -0.18571429 -0.17142857 -0.15714286 -0.14285714 -0.12857143 -0.11428571 -0.1 -0.08571429 -0.07142857 -0.05714286 -0.04285714 -0.02857143 -0.01428571 0 0 0 0 0 0
  line L9 (-18.5945, 25.9818) -> (-18.3983, 26.4277)
  arc A19 (-18.2674, 26.4793) -> (-18.3983, 26.4277) centre (-18.3068, 26.3874) ccw
  arc A20 (-18.2674, 26.4793) -> (-17.3108, 26.1163) centre (-13.5, 37.5997) ccw
  arc A21 (-17.2471, 25.9908) -> (-17.3108, 26.1163) centre (-17.3423, 26.0214) ccw
  line L10 (-17.2471, 25.9908) -> (-17.3961, 25.527)
  spline S10 degree 5 poles (-17.3961, 25.527) (-17.3978, 25.5216) (-17.4011, 25.5108) (-17.4057, 25.4944) (-17.4111, 25.4725) (-17.4167, 25.4447) (-17.4216, 25.4168) (-17.426, 25.3887) (-17.4301, 25.3605) (-17.434, 25.3322) (-17.4378, 25.304) (-17.4413, 25.2756) (-17.4445, 25.2472) (-17.4473, 25.2186) (-17.4498, 25.19) (-17.4519, 25.1613) (-17.4537, 25.1325) (-17.4553, 25.1036) (-17.4566, 25.0747) (-17.4578, 25.0458) (-17.4587, 25.0168) (-17.4594, 24.9877) (-17.4599, 24.9586) (-17.4601, 24.9294) (-17.4601, 24.9002) (-17.4599, 24.871) (-17.4595, 24.8417) (-17.4588, 24.8123) (-17.458, 24.7829) (-17.457, 24.7535) (-17.4558, 24.7241) (-17.4544, 24.6946) (-17.4527, 24.665) (-17.451, 24.6355) (-17.449, 24.6059) (-17.4468, 24.5762) (-17.4444, 24.5465) (-17.4419, 24.5168) (-17.4392, 24.4871) (-17.4363, 24.4574) (-17.4332, 24.4276) (-17.43, 24.3978) (-17.4266, 24.3679) (-17.423, 24.338) (-17.4193, 24.3081) (-17.4154, 24.2782) (-17.4113, 24.2483) (-17.407, 24.2183) (-17.4026, 24.1883) (-17.3981, 24.1583) (-17.3933, 24.1283) (-17.3884, 24.0983) (-17.3834, 24.0682) (-17.3782, 24.0381) (-17.3728, 24.008) (-17.3673, 23.9779) (-17.3616, 23.9477) (-17.3558, 23.9176) (-17.3498, 23.8874) (-17.3437, 23.8572) (-17.3374, 23.827) (-17.3309, 23.7968) (-17.3243, 23.7666) (-17.3176, 23.7364) (-17.3107, 23.7061) (-17.3037, 23.6759) (-17.2965, 23.6456) (-17.2892, 23.6153) (-17.2817, 23.585) (-17.2741, 23.5547) (-17.2663, 23.5244) (-17.26, 23.5001) (-17.2552, 23.4819) (-17.252, 23.4698) (-17.2503, 23.4638) knots 0 0 0 0 0 0 0.01428571 0.02857143 0.04285714 0.05714286 0.07142857 0.08571429 0.1 0.11428571 0.12857143 0.14285714 0.15714286 0.17142857 0.18571429 0.2 0.21428571 0.22857143 0.24285714 0.25714286 0.27142857 0.28571429 0.3 0.31428571 0.32857143 0.34285714 0.35714286 0.37142857 0.38571429 0.4 0.41428571 0.42857143 0.44285714 0.45714286 0.47142857 0.48571429 0.5 0.51428571 0.52857143 0.54285714 0.55714286 0.57142857 0.58571429 0.6 0.61428571 0.62857143 0.64285714 0.65714286 0.67142857 0.68571429 0.7 0.71428571 0.72857143 0.74285714 0.75714286 0.77142857 0.78571429 0.8 0.81428571 0.82857143 0.84285714 0.85714286 0.87142857 0.88571429 0.9 0.91428571 0.92857143 0.94285714 0.95714286 0.97142857 0.98571429 1 1 1 1 1 1
  arc A22 (-17.2503, 23.4638) -> (-16.467, 23.2788) centre (-13.5, 37.5997) ccw
  spline S11 degree 5 poles (-16.467, 23.2788) (-16.4628, 23.2835) (-16.4545, 23.2929) (-16.4421, 23.3071) (-16.4256, 23.3259) (-16.4051, 23.3496) (-16.3847, 23.3733) (-16.3645, 23.397) (-16.3444, 23.4208) (-16.3244, 23.4447) (-16.3046, 23.4686) (-16.2849, 23.4926) (-16.2654, 23.5166) (-16.246, 23.5407) (-16.2267, 23.5649) (-16.2076, 23.5891) (-16.1886, 23.6133) (-16.1697, 23.6376) (-16.151, 23.662) (-16.1325, 23.6864) (-16.1141, 23.7109) (-16.0958, 23.7354) (-16.0777, 23.76) (-16.0597, 23.7846) (-16.0419, 23.8093) (-16.0243, 23.834) (-16.0068, 23.8588) (-15.9894, 23.8837) (-15.9722, 23.9086) (-15.9552, 23.9335) (-15.9383, 23.9586) (-15.9216, 23.9836) (-15.905, 24.0087) (-15.8886, 24.0339) (-15.8724, 24.0591) (-15.8563, 24.0844) (-15.8404, 24.1097) (-15.8247, 24.1351) (-15.8092, 24.1605) (-15.7938, 24.186) (-15.7786, 24.2116) (-15.7636, 24.2372) (-15.7487, 24.2628) (-15.7341, 24.2885) (-15.7197, 24.3143) (-15.7054, 24.3401) (-15.6913, 24.3659) (-15.6774, 24.3918) (-15.6637, 24.4178) (-15.6502, 24.4438) (-15.637, 24.4699) (-15.6239, 24.496) (-15.6111, 24.5222) (-15.5985, 24.5484) (-15.5861, 24.5747) (-15.574, 24.6011) (-15.5621, 24.6275) (-15.5503, 24.654) (-15.5388, 24.6805) (-15.5276, 24.707) (-15.5166, 24.7337) (-15.506, 24.7604) (-15.4958, 24.7872) (-15.486, 24.814) (-15.4764, 24.841) (-15.4671, 24.868) (-15.458, 24.895) (-15.4491, 24.922) (-15.4405, 24.9491) (-15.4323, 24.9763) (-15.425, 25.0036) (-15.4199, 25.0257) (-15.4167, 25.0423) (-15.4149, 25.0535) (-15.414, 25.0591) knots -1 -1 -1 -1 -1 -1 -0.98571429 -0.97142857 -0.95714286 -0.94285714 -0.92857143 -0.91428571 -0.9 -0.88571429 -0.87142857 -0.85714286 -0.84285714 -0.82857143 -0.81428571 -0.8 -0.78571429 -0.77142857 -0.75714286 -0.74285714 -0.72857143 -0.71428571 -0.7 -0.68571429 -0.67142857 -0.65714286 -0.64285714 -0.62857143 -0.61428571 -0.6 -0.58571429 -0.57142857 -0.55714286 -0.54285714 -0.52857143 -0.51428571 -0.5 -0.48571429 -0.47142857 -0.45714286 -0.44285714 -0.42857143 -0.41428571 -0.4 -0.38571429 -0.37142857 -0.35714286 -0.34285714 -0.32857143 -0.31428571 -0.3 -0.28571429 -0.27142857 -0.25714286 -0.24285714 -0.22857143 -0.21428571 -0.2 -0.18571429 -0.17142857 -0.15714286 -0.14285714 -0.12857143 -0.11428571 -0.1 -0.08571429 -0.07142857 -0.05714286 -0.04285714 -0.02857143 -0.01428571 0 0 0 0 0 0
  line L11 (-15.414, 25.0591) -> (-15.3399, 25.5406)
  arc A23 (-15.2267, 25.6244) -> (-15.3399, 25.5406) centre (-15.241, 25.5254) ccw
  arc A24 (-15.2267, 25.6244) -> (-14.2088, 25.5213) centre (-13.5, 37.5997) ccw
  arc A25 (-14.1148, 25.4166) -> (-14.2088, 25.5213) centre (-14.2147, 25.4215) ccw
  line L12 (-14.1148, 25.4166) -> (-14.1386, 24.93)
  spline S12 degree 5 poles (-14.1386, 24.93) (-14.1389, 24.9243) (-14.1393, 24.913) (-14.1395, 24.896) (-14.139, 24.8734) (-14.1373, 24.8452) (-14.1348, 24.8169) (-14.1317, 24.7886) (-14.1284, 24.7604) (-14.1249, 24.7321) (-14.1212, 24.7038) (-14.1173, 24.6754) (-14.113, 24.6471) (-14.1084, 24.6188) (-14.1033, 24.5906) (-14.098, 24.5623) (-14.0923, 24.534) (-14.0863, 24.5057) (-14.0801, 24.4774) (-14.0737, 24.4492) (-14.0671, 24.4209) (-14.0603, 24.3927) (-14.0532, 24.3644) (-14.0459, 24.3362) (-14.0383, 24.308) (-14.0305, 24.2798) (-14.0225, 24.2516) (-14.0143, 24.2234) (-14.0059, 24.1953) (-13.9973, 24.1671) (-13.9885, 24.139) (-13.9795, 24.1108) (-13.9703, 24.0827) (-13.9609, 24.0546) (-13.9514, 24.0265) (-13.9416, 23.9985) (-13.9316, 23.9704) (-13.9215, 23.9424) (-13.9112, 23.9144) (-13.9007, 23.8864) (-13.89, 23.8584) (-13.8792, 23.8304) (-13.8682, 23.8025) (-13.857, 23.7746) (-13.8456, 23.7467) (-13.8341, 23.7188) (-13.8224, 23.6909) (-13.8105, 23.6631) (-13.7985, 23.6352) (-13.7863, 23.6074) (-13.774, 23.5797) (-13.7615, 23.5519) (-13.7488, 23.5242) (-13.736, 23.4965) (-13.723, 23.4688) (-13.7099, 23.4411) (-13.6966, 23.4135) (-13.6832, 23.3858) (-13.6696, 23.3583) (-13.6559, 23.3307) (-13.642, 23.3031) (-13.6279, 23.2756) (-13.6138, 23.2481) (-13.5994, 23.2207) (-13.5849, 23.1932) (-13.5703, 23.1658) (-13.5555, 23.1384) (-13.5406, 23.1111) (-13.5256, 23.0838) (-13.5104, 23.0565) (-13.495, 23.0292) (-13.4827, 23.0074) (-13.4733, 22.9911) (-13.467, 22.9802) (-13.4639, 22.9748) knots 0 0 0 0 0 0 0.01428571 0.02857143 0.04285714 0.05714286 0.07142857 0.08571429 0.1 0.11428571 0.12857143 0.14285714 0.15714286 0.17142857 0.18571429 0.2 0.21428571 0.22857143 0.24285714 0.25714286 0.27142857 0.28571429 0.3 0.31428571 0.32857143 0.34285714 0.35714286 0.37142857 0.38571429 0.4 0.41428571 0.42857143 0.44285714 0.45714286 0.47142857 0.48571429 0.5 0.51428571 0.52857143 0.54285714 0.55714286 0.57142857 0.58571429 0.6 0.61428571 0.62857143 0.64285714 0.65714286 0.67142857 0.68571429 0.7 0.71428571 0.72857143 0.74285714 0.75714286 0.77142857 0.78571429 0.8 0.81428571 0.82857143 0.84285714 0.85714286 0.87142857 0.88571429 0.9 0.91428571 0.92857143 0.94285714 0.95714286 0.97142857 0.98571429 1 1 1 1 1 1
  arc A26 (-13.4639, 22.9748) -> (-12.6594, 22.9989) centre (-13.5, 37.5997) ccw
  spline S13 degree 5 poles (-12.6594, 22.9989) (-12.6566, 23.0045) (-12.651, 23.0158) (-12.6426, 23.0326) (-12.6316, 23.0551) (-12.6179, 23.0832) (-12.6043, 23.1114) (-12.5909, 23.1396) (-12.5777, 23.1678) (-12.5646, 23.196) (-12.5516, 23.2242) (-12.5388, 23.2525) (-12.5262, 23.2808) (-12.5137, 23.3091) (-12.5013, 23.3374) (-12.4891, 23.3657) (-12.477, 23.394) (-12.4651, 23.4224) (-12.4534, 23.4508) (-12.4417, 23.4791) (-12.4303, 23.5075) (-12.419, 23.536) (-12.4079, 23.5644) (-12.3969, 23.5928) (-12.3861, 23.6213) (-12.3754, 23.6498) (-12.3649, 23.6783) (-12.3546, 23.7067) (-12.3444, 23.7352) (-12.3344, 23.7638) (-12.3246, 23.7923) (-12.3149, 23.8208) (-12.3054, 23.8494) (-12.2961, 23.8779) (-12.287, 23.9065) (-12.278, 23.9351) (-12.2692, 23.9636) (-12.2606, 23.9922) (-12.2522, 24.0208) (-12.2439, 24.0494) (-12.2358, 24.078) (-12.228, 24.1066) (-12.2203, 24.1352) (-12.2128, 24.1638) (-12.2055, 24.1925) (-12.1984, 24.2211) (-12.1915, 24.2497) (-12.1848, 24.2783) (-12.1783, 24.3069) (-12.172, 24.3356) (-12.1659, 24.3642) (-12.1601, 24.3928) (-12.1544, 24.4214) (-12.1491, 24.45) (-12.144, 24.4786) (-12.139, 24.5072) (-12.1343, 24.5358) (-12.1299, 24.5644) (-12.1256, 24.593) (-12.1216, 24.6216) (-12.1179, 24.6501) (-12.1146, 24.6787) (-12.1117, 24.7072) (-12.1091, 24.7357) (-12.1069, 24.7642) (-12.1049, 24.7927) (-12.1031, 24.8211) (-12.1015, 24.8495) (-12.1001, 24.878) (-12.0993, 24.9063) (-12.0993, 24.9346) (-12.1001, 24.9572) (-12.1013, 24.9741) (-12.1024, 24.9854) (-12.103, 24.991) knots -1 -1 -1 -1 -1 -1 -0.98571429 -0.97142857 -0.95714286 -0.94285714 -0.92857143 -0.91428571 -0.9 -0.88571429 -0.87142857 -0.85714286 -0.84285714 -0.82857143 -0.81428571 -0.8 -0.78571429 -0.77142857 -0.75714286 -0.74285714 -0.72857143 -0.71428571 -0.7 -0.68571429 -0.67142857 -0.65714286 -0.64285714 -0.62857143 -0.61428571 -0.6 -0.58571429 -0.57142857 -0.55714286 -0.54285714 -0.52857143 -0.51428571 -0.5 -0.48571429 -0.47142857 -0.45714286 -0.44285714 -0.42857143 -0.41428571 -0.4 -0.38571429 -0.37142857 -0.35714286 -0.34285714 -0.32857143 -0.31428571 -0.3 -0.28571429 -0.27142857 -0.25714286 -0.24285714 -0.22857143 -0.21428571 -0.2 -0.18571429 -0.17142857 -0.15714286 -0.14285714 -0.12857143 -0.11428571 -0.1 -0.08571429 -0.07142857 -0.05714286 -0.04285714 -0.02857143 -0.01428571 0 0 0 0 0 0
  line L13 (-12.103, 24.991) -> (-12.156, 25.4753)